Wheel (Autodesk Fusion 360 design; units mm, degrees)
Autodesk Fusion 360 part; units mm, degrees
note: some values were not read from the file. Set by a fixed rule: which face or edge a step refers to.
sketch "Sketch1" plane through (0, 0, 0) normal (0, 0, 1) x (1, 0, 0)
  circle A0 centre (0, 0) radius 62
  circle A1 centre (0, 0) radius 65
  circle A2 centre (0, 0) radius 60
  line L0 (-6.2, 3.5796) -> (-6.2, -3.5796)
  line L1 (-6.2, -3.5796) -> (0, -7.1591)
  line L2 (0, -7.1591) -> (6.2, -3.5796)
  line L3 (6.2, -3.5796) -> (6.2, 3.5796)
  line L4 (6.2, 3.5796) -> (0, 7.1591)
  line L5 (0, 7.1591) -> (-6.2, 3.5796)
  circle A3 centre (0, 0) radius 12
  dimension "d1" = 124
  dimension "d2" = 3
  dimension "d6" = -2
  dimension "d10" = 12.4
  dimension "d11" = 24
  constraint coincident A0.centre A1.centre
  measures "d1" diameter of A0
  measures "d10" distance of L0.start L3.end
  measures "d11" diameter of A3
extrude "Extrude1" add sketch "Sketch1" along normal blind 60 contours A1 makes body 1
fillet "Fillet1" radius 65 2 edges at (-60.6013, -23.505, 0) (-60.6013, -23.505, 60) on bodies 1
extrude "Extrude2" add sketch "Sketch1" along normal blind 60 contours A0 bodies 1
extrude "Extrude3" add sketch "Sketch1" along normal blind 45 separate body contours L0 L1 L2 L3 L4 L5 | A3 makes body 2
extrude "Extrude6" cut sketch "Sketch1" along normal blind 20 contours L0 L1 L2 L3 L4 L5 bodies 2
sketch "Sketch4" plane through (0, 0, 45) normal (0, 0, 1) x (-1, 0, 0)
  circle A0 centre (0, 0) radius 12
  circle A1 centre (0, 0) radius 9
  circle A2 centre (0, 0) radius 2.25
  dimension "d24" = 18
  dimension "d27" = 4.5
  constraint coincident A0.centre A1.centre
  constraint concentric A0 A2
  measures "d24" diameter of A1
  measures "d27" diameter of A2
extrude "Extrude7" cut sketch "Sketch4" against normal blind 23 contours A1 | A2 bodies 2
extrude "Extrude8" cut sketch "Sketch4" against normal through all contours A2 bodies 2
split "Split1" by plane through (0, 0, 0) normal (1, 0, 0) bodies 2 1 makes body 4 at (59.932, -2.8549, 40) makes body 3 at (1.1407, 11.9457, 30)
sketch "Sketch3" plane through (0, 0, 0) normal (1, 0, 0) x (0, 1, 0)
  line L0 (12, 0) -> (12, 45)
  line L1 (60, 60) -> (60, 0)
  spline S0 degree 2 poles (60, 42.7084) (38.6783, 72.0378) (12, 45) knots 0 0 0 5.745728 5.745728 5.745728 weights 1 1.255877 1
  spline S1 degree 5 poles (12, 0) (12.0736, 1.4072) (12.2257, 4.1703) (12.4683, 8.1605) (12.8208, 13.1712) (13.313, 18.9163) (13.8663, 24.1439) (14.4994, 28.8619) (15.2424, 33.0896) (16.1409, 36.8626) (17.2571, 40.2342) (18.6633, 43.2616) (20.4363, 45.9935) (22.6524, 48.4596) (25.378, 50.6515) (28.6539, 52.4906) (32.483, 53.8021) (36.8108, 54.278) (41.5157, 53.5619) (46.3581, 51.4127) (51.0211, 47.7458) (54.9298, 42.947) (57.7005, 37.4294) (59.3453, 31.318) (60.0595, 24.6384) (60.1751, 17.3078) (60.0711, 10.8293) (60.0129, 5.5748) (60, 1.8888) (60, 0) knots 0 0 0 0 0 0 0.04 0.08 0.12 0.16 0.2 0.24 0.28 0.32 0.36 0.4 0.44 0.48 0.52 0.56 0.6 0.64 0.68 0.72 0.76 0.8 0.84 0.88 0.92 0.96 1 1 1 1 1 1
  line L2 (43.1085, 54.8385) -> (57.8548, 40.7724)
  line L3 (12, 0) -> (60, 0)
  line L4 (60, 0) -> (60, 10)
  line L5 (60, 10) -> (12, 10)
  line L6 (12, 10) -> (12, 0)
  line L7 (60, 15.024) -> (60, -15.024)
  point P0 (15.0944, 32.0363)
  point P1 (19.6548, 44.6752)
  point P2 (29.4272, 52.6234)
  point P3 (50.4816, 47.8054)
  dimension "d19" = 10
  constraint coincident L1 S0.start
  constraint coincident L0.end S0.end
  constraint coincident L0.start S1.start
  constraint midpoint P3 L2
  constraint horizontal L3
  constraint vertical L4
  constraint horizontal L5
  constraint vertical L6
  constraint coincident L1 L4.end
  constraint coincident L1.end S1.end
  constraint midpoint L1.end L7
  constraint coincident L1 L7.start
  measures "d19" distance of L0.start L5.end
extrude "Extrude4" add sketch "Sketch3" along normal mid plane 4 separate body contours L0 S1 L5 L6 | L1 S1 L3 L4 L5 L7 | L0 L1 S0 S1 L5 makes body 5
extrude "Extrude5" add 4 faces at (1.3333, 12, 3.3333) (0.6667, 12, 21.6667) (-1.3333, 12, 3.3333) (-0.6667, 12, 21.6667) along direction (0, -1, 0) blind 2 on bodies 5 bodies 5
pattern_circular "C-Pattern1" count 6 over 360 about axis through (0, 0, 1.75) along (0, 0, 1) of bodies 5 makes body 6 at (-25.4244, 12.3694, 3.3333) makes body 7 at (-25.4244, -12.3694, 3.3333) makes body 8 at (-2, -28.2028, 3.3333) makes body 9 at (23.4244, -15.8335, 3.3333) makes body 10 at (25.4244, 12.3694, 3.3333)
combine "Combine1" operation add target body 1 tool bodies 2 3 4 5 6 7 8 9 10
split "Split2" [suppressed]
ref_plane "WorkPlane1" through (6.2, 0, 22.5) normal (0.573576, 0.819152, 0) x (0, 0, 1)
split "Split3" [suppressed]
